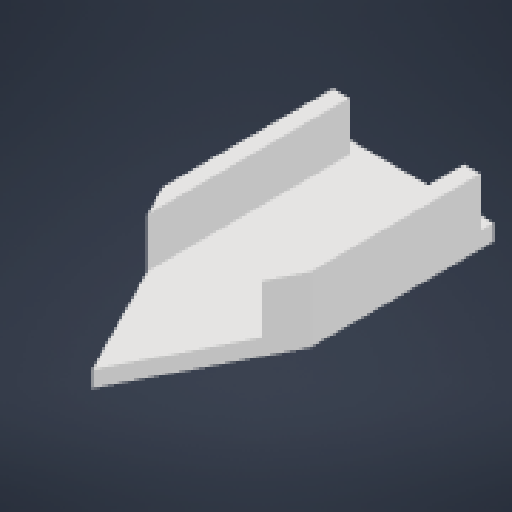
# Autodesk Inventor part: middleslide2
Saved by Autodesk Inventor 2026.2 (Build 302298000, 298)
## iProperties
Created: 2026-02-23
Part Number: middleslide2
Material: Generic
Document SubType Name: Sheet Metal
Designer: danda
Density: 1 g/cm^3
Sheet Metal Rule: Default_mm
Appearance: Default
Author: danda
Autodesk Inventor part; units mm, degrees
ref_plane "YZ Plane" through (0, 0, 0) normal (1, 0, 0) x (0, 1, 0)
ref_plane "XZ Plane" through (0, 0, 0) normal (0, 1, 0) x (-1, 0, 0)
ref_plane "XY Plane" through (0, 0, 0) normal (0, 0, 1) x (1, 0, 0)
sketch "Sketch1" plane through (0, 0, 0) normal (0, 0, 1) x (1, 0, 0)
  line L0 (10.7104, 9.7791) -> (45.7104, 9.7791)
  line L1 (45.7104, 9.7791) -> (45.7104, 24.7791)
  line L2 (10.7104, 9.7791) -> (10.7104, 24.7791)
  line L3 (5.7104, 24.7791) -> (5.7104, 4.7791)
  line L4 (5.7104, 4.7791) -> (50.7104, 4.7791)
  line L5 (50.7104, 4.7791) -> (50.7104, 24.7791)
  line L6 (5.7104, 24.7791) -> (10.7104, 24.7791)
  line L7 (45.7104, 24.7791) -> (50.7104, 24.7791)
  point P0 (0, 0)
  point P1 (28.2104, 9.7791)
  dimension "d0" = 35
  dimension "d1" = 15
  dimension "d2" = 15
  dimension "d29" = 5
  constraints: 16 end point, 3 horizontal, 2 perpendicular, 1 midpoint, 1 vertical, 2 other
  measures "d0" distance of L0.start L0.end
  measures "d1" distance of L0.end L1.end
  measures "d2" distance of L0.start L2.end
  measures "d29" distance from line of L4 point (28.21, 9.779)
extrude "Extrusion1" add sketch "Sketch1" along normal blind 100
sketch "Sketch3" plane through (10.7104, 9.7791, 0) normal (0, 1, 0) x (1, 0, 0)
  line L0 (-5, -100) -> (40, -100) projected
  line L1 (-5, 0) -> (-5, -100) projected
  line L2 (17.5, -100) -> (37.1919, -100) construction
  line L3 (-5, -85.7353) -> (-5, -100)
  line L4 (-5, -100) -> (17.5, -100)
  line L5 (40, 0) -> (40, -100) projected
  line L6 (17.5, -100) -> (37.1919, -100) construction
  line L7 (40, -85.7353) -> (40, -100)
  line L8 (40, -100) -> (17.5, -100)
  line L9 (40, 0) -> (40, -100) projected
  line L10 (17.5, -100) -> (-5, -36.462)
  line L11 (17.5, -100) -> (40, -36.462)
  line L12 (-5, -36.462) -> (40, -36.462)
  line L13 (35, 0) -> (35, -100) projected
  line L14 (0, 0) -> (0, -100) projected
  point P0 (-10.7104, 0)
  point P1 (-5, -77.7514)
  point P2 (40, -36.462)
  point P3 (-5, -60.8533)
  dimension "d33" = 39
  constraints: 18 end point, 6 point on line, 3 collinear, 3 horizontal, 1 midpoint, 1 perpendicular
  measures "d33" angle of L11 L10
extrude "Extrusion5" cut sketch "Sketch3" along normal through all both and the other way through all contours L1 L10 L14 L0 | L14 L10 L0 | L11 L13 L0 | L13 L11 L5 L0
sketch "Sketch4" plane through (50.7104, 4.7791, 0) normal (1, 0, 0) x (0, 0, -1)
  line L0 (0, 20) -> (-50.5815, 20) projected
  line L1 (0, 20) -> (-4, 20)
  line L2 (-4, 20) -> (-4, 5)
  line L3 (0, 5) -> (-50.5815, 5) projected
  line L4 (0, 20) -> (0, 5) projected
  line L5 (0, 5) -> (0, 20)
  line L6 (0, 20) -> (0, 5)
  line L7 (-4, 5) -> (0, 5)
  point P0 (0, -4.7791)
  dimension "d24" = 4
  constraints: 10 end point, 2 collinear, 2 perpendicular, 2 point on line
  measures "d24" distance of L0.start L1.end
extrude "Extrusion6" cut sketch "Sketch4" against normal through all
equation "\"BendRadius\" = Thickness"
equation "\"BendReliefWidth\" = Thickness"
equation "\"BendReliefDepth\" = 0.5 * Thickness"
equation "\"CornerReliefSize\" = 4 * Thickness"
equation "\"MinimumRemnant\" = 2 * Thickness"
equation "\"TransitionRadius\" = BendRadius"
equation "\"JacobiRadiusSize\" = BendRadius"
equation "\"GapSize\" = Thickness"
equation "\"Thickness\" = 0.5"
body "Solid1"
